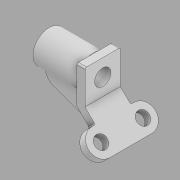
# Autodesk Inventor part: LAB7
Saved by Autodesk Inventor 2020 (Build 240168000, 168)
## iProperties
Created: 2019-09-26
Part Number: LAB7
Material: Genérico
Document SubType Name: Modeling
Designer: gerar
Density: 1 g/cm^3
Appearance: Valor por defecto
Author: gerar
Autodesk Inventor part; units mm, degrees
ref_plane "YZ Plane" through (0, 0, 0) normal (1, 0, 0) x (0, 1, 0)
ref_plane "XZ Plane" through (0, 0, 0) normal (0, 1, 0) x (-1, 0, 0)
ref_plane "XY Plane" through (0, 0, 0) normal (0, 0, 1) x (1, 0, 0)
sketch "Boceto1" plane through (0, 0, 0) normal (0, 0, 1) x (1, 0, 0)
  line L0 (0, 67) -> (16, 67)
  line L1 (16, 67) -> (16, 0)
  line L2 (16, 0) -> (71.6777, -55.6777)
  line L3 (71.6777, -55.6777) -> (60.364, -66.9914)
  line L4 (60.364, -66.9914) -> (0, -6.6274)
  line L5 (0, -6.6274) -> (0, 67)
  line L6 (-57.0485, 0) -> (121.2498, 0) construction
  line L7 (0, -93.7897) -> (0, 93.7983) construction
  line L8 (-31.5773, 32) -> (95.7786, 32) construction
  line L9 (42.2994, 0) -> (47.9017, 5.6023) construction
  line L10 (-3.3802, -38.7017) -> (0, -35.3215) construction
  line L11 (42.6863, -49.3137) -> (54, -38) construction
  point P0 (0, 0)
  dimension "d0" = 16
  dimension "d3" = 35
  dimension "d6" = 25
  dimension "d7" = 70
  dimension "d10" = 45
  dimension "d11" = 0
  dimension "d44" = 45
  dimension "d46" = 32
  constraints: 20 end point, 4 parallel, 4 point on line, 3 perpendicular, 2 horizontal, 1 collinear, 1 equal length
  measures "d0" distance of L0.start L0.end
  measures "d3" distance between parallel lines of L8 L0
  measures "d6" distance between parallel lines of L3 L11
  measures "d7" distance from line of L11.end L8
  measures "d10" angle of L6 L3
  measures "d11" distance from line of L1.end L6
  measures "d44" angle of L4 L7
  measures "d46" distance from line of L1.end L8
extrude "Extrusión1" add sketch "Boceto1" along normal mid plane 70
sketch "Boceto2" plane through (16, 0, -35) normal (1, 0, 0) x (0, 0, -1)
  line L0 (0, 67) -> (0, 0) construction
  line L1 (0, 67) -> (-70, 67) construction
  line L2 (-70, 0) -> (-70, 67) construction
  line L3 (0, 0) -> (-70, 0) construction
  circle A0 centre (-35, 33.5) radius 32
  point P0 (-35, 0)
  dimension "d14" = 64
  constraints: 1 centre point
  measures "d14" diameter of A0
extrude "Extrusión2" add sketch "Boceto2" against normal blind 106
sketch "Boceto3" plane through (16, 0, -35) normal (0.7071068, 0.7071068, 0) x (-0.7071068, 0.7071068, 0)
  line L0 (-53.7401, 76.5) -> (-53.7401, -6.5) construction
  line L1 (-28.7401, 76.5) -> (-28.7401, -6.5)
  line L2 (-78.7401, -6.5) -> (-78.7401, 76.5)
  arc A0 (-28.7401, 76.5) -> (-78.7401, 76.5) centre (-53.7401, 76.5) ccw
  arc A1 (-78.7401, -6.5) -> (-28.7401, -6.5) centre (-53.7401, -6.5) ccw
  line L3 (-78.7401, 0) -> (-78.7401, 70) projected
  line L4 (-78.7401, 35) -> (0, 35) construction
  line L5 (0, 0) -> (0, 70) construction
  point P0 (11.3137, 35)
  point P1 (-53.7401, 35)
  dimension "d17" = 83
  dimension "d18" = 41.5
  dimension "d19" = 25
  constraints: 10 end point, 4 point on circle, 4 tangent, 3 midpoint, 2 centre point, 1 collinear, 1 parallel, 1 vertical
  measures "d17" distance of L0.end L0.start
  measures "d18" distance from line of L4 L0.end
  measures "d19" radius of A1
extrude "Extrusión3" add sketch "Boceto3" against normal up to surface (16 mm away)
sketch "Boceto4" plane through (0, 0, 0) normal (0, 0, 1) x (1, 0, 0)
  line L0 (-73.6419, -21.9588) -> (52.9945, -68.6101)
  line L1 (-90, 65.5) -> (-90, 1.5) projected
  arc A0 (-90, 1.5) -> (-73.6419, -21.9588) centre (-65, 1.5) ccw
  arc A1 (52.9945, -68.6101) -> (60.364, -66.9914) centre (55.4142, -62.0416) ccw
  line L2 (-90, 65.5) -> (-90, 1.5) construction
  line L3 (0, 1.5) -> (0, 65.5) construction
  line L4 (71.6777, -55.6777) -> (60.364, -66.9914) construction
  line L5 (-90, 65.5) -> (-90, 1.5) construction
  line L6 (0, 1.5) -> (-90, 1.5) construction
  line L7 (0, 67) -> (0, -6.6274) construction
  line L8 (0, -6.6274) -> (25.0086, -31.636) construction
  line L9 (60.364, -66.9914) -> (25.0086, -31.636) construction
  line L10 (0, 1.5) -> (-90, 1.5) projected
  line L11 (25.0086, -31.636) -> (60.364, -66.9914) construction
  line L12 (71.6777, -55.6777) -> (60.364, -66.9914) construction
  line L13 (36.3223, -20.3223) -> (71.6777, -55.6777) construction
  line L14 (36.3223, -20.3223) -> (25.0086, -31.636) construction
  line L15 (-90, 1.5) -> (0, 1.5)
  line L16 (0, 0) -> (0, -6.6274)
  line L17 (0, -6.6274) -> (60.364, -66.9914)
  line L18 (25.0086, -31.636) -> (0, -6.6274) projected
  dimension "d22" = 25
  dimension "d23" = 7
  constraints: 8 end point, 4 point on circle, 4 tangent, 2 centre point, 2 collinear, 1 perpendicular
  measures "d22" radius of A0
  measures "d23" radius of A1
extrude "Nervio1" add sketch "Boceto4" along normal mid plane 16 rib yes fills toward (-85.4657, -12.7709) open curves A0 L0 A1
sketch "Boceto5" plane through (16, 0, 35) normal (1, 0, 0) x (0, 0, -1)
  arc A0 (43, 2.5161) -> (27, 2.5161) centre (35, 33.5) ccw projected
  point P0 (35, 0)
  constraints: 1 coincident
hole "Agujero1" at (16, 33.5, 0) direction (-1, 0, 0) diameter 32 end through all
sketch "Boceto6" plane through (16, 0, -35) normal (0.7071068, 0.7071068, 0) x (-0.7071068, 0.7071068, 0)
  arc A0 (-28.7401, 76.5) -> (-78.7401, 76.5) centre (-53.7401, 76.5) ccw projected
  arc A1 (-78.7401, -6.5) -> (-28.7401, -6.5) centre (-53.7401, -6.5) ccw projected
  point P0 (11.3137, 35)
  point P1 (-53.7401, -6.5)
  constraints: 2 coincident
hole "Agujero2" at (54, -38, 41.5) at (54, -38, -41.5) direction (-0.7071068, -0.7071068, 0) diameter 25 end through all
fillet "Empalme1" radius 3 7 edges at (8, 67, 35) (8, 67, -35) (30.6655, -25.9792, 35) (30.6655, -25.9792, -35) (-45.0002, 2.5161, -8) (0, 65.5, 0) (-45.0002, 2.5161, 8)
equation "\"d18\" = 0.5 * d17"
